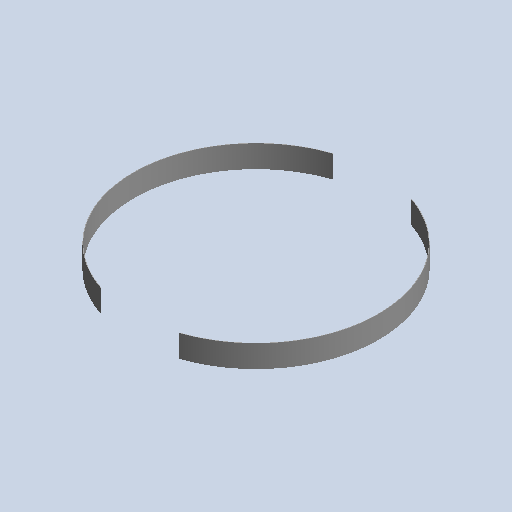
# Autodesk Inventor part: Enclosure
Saved by Autodesk Inventor 2026 (Build 300175050, 175E)
## iProperties
Part Number: Enclosure
Material: Generic
Document SubType Name: Modeling
Designer: Kartik
Mass: 43.7673 g
Surface Area: 898.917 cm^2
Volume: 43.7673 cm^3
Density: 1 g/cm^3
Appearance: Default
Author: Kartik
Autodesk Inventor part; units mm, degrees
ref_plane "YZ Plane" through (0, 0, 0) normal (1, 0, 0) x (0, 1, 0)
ref_plane "XZ Plane" through (0, 0, 0) normal (0, 1, 0) x (-1, 0, 0)
ref_plane "XY Plane" through (0, 0, 0) normal (0, 0, 1) x (1, 0, 0)
sketch "Sketch1" plane through (0, 0, 0) normal (0, 1, 0) x (-1, 0, 0)
  line L0 (-70, -252.7863) -> (70, -252.7863)
  arc A0 (-70, 207.5114) -> (-70, -207.5114) centre (0, 0) ccw
  arc A1 (70, -207.5114) -> (70, 207.5114) centre (0, 0) ccw
  arc A2 (-70, 208.5665) -> (-70, -208.5665) centre (0, 0) ccw
  arc A3 (70, -208.5665) -> (70, 208.5665) centre (0, 0) ccw
  line L1 (70, -208.5665) -> (70, -207.5114)
  line L2 (70, 207.5114) -> (70, 208.5665)
  line L3 (-70, 208.5665) -> (-70, 207.5114)
  line L4 (-70, -207.5114) -> (-70, -208.5665)
  dimension "d2" = 140
  constraints: 10 end point, 8 point on circle, 4 centre point, 4 parallel, 1 coincident
  measures "d2" distance of L0.start L0.end
extrude "Extrusion1" add sketch "Sketch1" along normal blind 40
body "Solid1"
